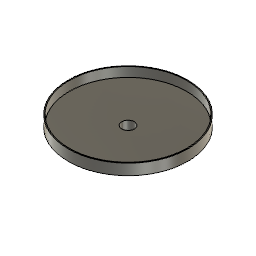
Sprocket Case (Autodesk Fusion 360 design; units mm, degrees)
Autodesk Fusion 360 part; units mm, degrees
sketch "Sketch1" plane through (0, 0, 0) normal (0, 0, 1) x (1, 0, 0)
  circle A0 centre (0, 0) radius 118.11
  circle A1 centre (0, 0) radius 120.11
  line L0 (120.11, 0) -> (-120.11, 0)
  dimension "d1" = 236.22
  dimension "d2" = 240.22
  constraint coincident A0.centre A1.centre
  constraint concentric A0 A1
  constraint midpoint L0 A0.centre
  constraint coincident A1 L0.end
  constraint horizontal L0
  measures "d1" diameter of A0
  measures "d2" diameter of A1
extrude "Extrude1" add sketch "Sketch1" along normal blind 22.05 contours A0 A1 L0 | A0 A1 L0 makes body 1
extrude "Extrude2" add sketch "Sketch1" along normal blind 3 contours A0 L0 | A0 L0 bodies 1
sketch "Sketch2" plane through (0, 0, 3) normal (0, 0, 1) x (-1, 0, 0)
  circle A0 centre (0, 0) radius 12.7
  circle A1 centre (0, 0) radius 118.11
  dimension "d7" = 25.4
  constraint coincident A0.centre A1.centre
  measures "d7" diameter of A0
extrude "Extrude3" cut sketch "Sketch2" against normal blind 3 contours A0 bodies 1
sketch "Sketch3" plane through (0, 0, 0) normal (0, 0, 1) x (1, 0, 0)
  circle A0 centre (0, 0) radius 12.7
  circle A1 centre (0, 0) radius 14.7
  line L0 (3.175, 0) -> (-3.175, 0)
  line L1 (0, 0) -> (0, -14.54)
  line L2 (-3.175, 0) -> (3.175, 0)
  line L3 (3.175, 0) -> (3.175, -14.54)
  line L4 (3.175, -14.54) -> (-3.175, -14.54)
  line L5 (-3.175, -14.54) -> (-3.175, 0)
  line L6 (4.175, 0) -> (-4.175, 0)
  line L7 (-4.175, 0) -> (4.175, 0)
  line L8 (4.175, 0) -> (4.175, -15.54)
  line L9 (4.175, -15.54) -> (-4.175, -15.54)
  line L10 (-4.175, -15.54) -> (-4.175, 0)
  dimension "d10" = 25.4
  dimension "d11" = 29.4
  dimension "d14" = 6.35
  dimension "d16" = 14.54
  dimension "d17" = 14.54
  dimension "d18" = 8.35
  dimension "d19" = 15.54
  constraint coincident A0.centre A1.centre
  constraint midpoint L0 A0.centre
  constraint horizontal L0
  constraint perpendicular L0 L1
  constraint horizontal L2
  constraint vertical L3
  constraint horizontal L4
  constraint vertical L5
  constraint midpoint A0.centre L6
  constraint perpendicular L5 L6
  constraint horizontal L7
  constraint vertical L8
  constraint horizontal L9
  constraint vertical L10
  measures "d10" diameter of A0
  measures "d11" diameter of A1
  measures "d14" distance of L0.start L0.end
  measures "d16" distance of A0.centre L1.end
  measures "d17" distance of L0.end L4.end
  measures "d18" distance of L6.start L6.end
  measures "d19" distance of L6.end L9.end
extrude "Extrude4" add sketch "Sketch3" against normal blind 25.4 separate body contours A0 A1 L8 L10 | A0 A1 L5 L10 | A0 A1 L3 L8 | A0 A1 L1 L4 L5 | A0 A1 L1 L3 L4 | A1 L4 makes body 2
extrude "Extrude5" cut sketch "Sketch3" against normal blind 25.4 contours A0 A1 L1 L4 L5 | A0 A1 L1 L3 L4 | A1 L4 L5 | A1 L3 L4 bodies 2 makes body 3 at (7.9025, -12.3952, -16.9333)
extrude "Extrude6" add sketch "Sketch3" against normal blind 25.4 contours A1 L3 L4 L5 L8 L9 L10 bodies 1 2 3
